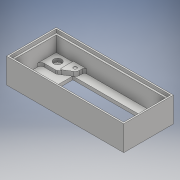
# Autodesk Inventor part: top
Saved by Autodesk Inventor 2018 (Build 220112000, 112)
## iProperties
Created: 2018-01-10
Part Number: top
Material: Generic
Document SubType Name: Modeling
Designer: gregg
Density: 1 g/cm^3
Appearance: Default
Author: gregg
Autodesk Inventor part; units mm, degrees
ref_plane "YZ Plane" through (0, 0, 0) normal (1, 0, 0) x (0, 1, 0)
ref_plane "XZ Plane" through (0, 0, 0) normal (0, 1, 0) x (-1, 0, 0)
ref_plane "XY Plane" through (0, 0, 0) normal (0, 0, 1) x (1, 0, 0)
sketch "Sketch1" plane through (0, 0, 0) normal (0, 0, 1) x (1, 0, 0)
  line L0 (0, 0) -> (100, 0)
  line L1 (100, 0) -> (100, 39)
  line L2 (100, 39) -> (0, 39)
  line L3 (0, 39) -> (0, 0)
  dimension "d45" = 100
  dimension "d46" = 39
  constraints: 8 end point, 2 parallel, 1 horizontal, 1 perpendicular
  measures "d45" distance of L1.end L2.end
  measures "d46" distance of L2.end L0.start
extrude "bottom" add sketch "Sketch1" along normal blind 3
sketch "Sketch5" plane through (0, 0, 0) normal (0, 0, -1) x (-1, 0, 0)
  line L0 (0, 0) -> (-100, 0) projected
  line L1 (0, 39) -> (0, 0) projected
  line L2 (-100, 39) -> (0, 39) projected
  line L3 (-100, 0) -> (-100, 39) projected
  line L4 (3, 42) -> (3, -3)
  line L5 (3, -3) -> (-103, -3)
  line L6 (-103, -3) -> (-103, 42)
  line L7 (-103, 42) -> (3, 42)
  dimension "d30" = 3
  constraints: 8 end point, 3 other
  measures "d30" distance between parallel lines of L2 L7
extrude "walls" add sketch "Sketch5" against normal blind 19.6
sketch "holes" plane through (0, 0, 0) normal (0, 0, 1) x (1, 0, 0)
  line L0 (0, 0) -> (100, 0) projected
  line L1 (100, 0) -> (100, 39) projected
  line L2 (100, 39) -> (0, 39) projected
  line L3 (0, 39) -> (0, 0) projected
  circle A0 centre (21.5, 34.5) radius 1.55 construction
  circle A1 centre (96.5, 34.5) radius 1.55 construction
  circle A2 centre (96.5, 3.5) radius 1.55 construction
  circle A3 centre (21.5, 3.5) radius 1.55 construction
  line L4 (21.5, 34.5) -> (21.5, 3.5) construction
  line L5 (21.5, 3.5) -> (96.5, 3.5) construction
  line L6 (96.5, 3.5) -> (96.5, 34.5) construction
  line L7 (96.5, 34.5) -> (21.5, 34.5) construction
  dimension "d33" = 3.1
  dimension "d34" = 75
  dimension "d35" = 31
  dimension "d50" = 3.5
  dimension "d51" = 3.5
  constraints: 8 end point, 4 centre point, 3 equal radius, 2 horizontal, 2 vertical
  measures "d33" diameter of A0
  measures "d34" distance of L6.end L4.start
  measures "d35" distance of L4.end L4.start
  measures "d50" distance from line of L1 L5.end
  measures "d51" distance from line of L0 L5.end
sketch "Sketch8" plane through (0, 0, 0) normal (0, 0, -1) x (-1, 0, 0)
  line L0 (-95, 6.3) -> (-23, 6.3)
  line L1 (-23, 6.3) -> (-23, 31)
  line L2 (-23, 31) -> (-95, 31)
  line L3 (-95, 31) -> (-95, 6.3)
  line L4 (3, -3) -> (-103, -3) projected
  line L5 (-96.5, 3.5) -> (-96.5, 34.5) construction
  line L6 (-21.5, 34.5) -> (-21.5, 3.5) construction
  point P0 (0, 0)
  dimension "d99" = 1.5
  dimension "d100" = 1.5
  dimension "d101" = 3.5
  dimension "d102" = 2.8
  constraints: 8 end point, 2 parallel, 1 horizontal, 1 perpendicular
  measures "d99" distance between parallel lines of L5 L3
  measures "d100" distance between parallel lines of L6 L1
  measures "d101" distance from line of L2 L5.end
  measures "d102" distance from line of L0 L5.start
extrude "display" cut sketch "Sketch8" along normal through all both and the other way through all
sketch "Sketch7" plane through (0, 0, 3) normal (0, 0, 1) x (1, 0, 0)
  circle A0 centre (96.5, 34.5) radius 1.55 construction
  circle A1 centre (21.5, 3.5) radius 1.55 construction
  circle A2 centre (21.5, 34.5) radius 1.55 construction
  arc A3 (23.4365, 31) -> (25.5, 34.5) centre (21.5, 34.5) ccw
  line L0 (15.5, 39) -> (27.5, 39)
  line L1 (0, 39) -> (100, 39) projected
  arc A4 (27.5, 39) -> (25.5, 37) centre (27.5, 37) ccw
  line L2 (25.5, 37) -> (25.5, 34.5)
  line L3 (16.3235, 0) -> (26.6765, 0)
  line L4 (23, 31) -> (95, 31) construction
  arc A5 (92.6921, 34.5) -> (96.7797, 30.7024) centre (96.5, 34.5) ccw
  line L5 (92.6921, 34.5) -> (92.6921, 36)
  arc A6 (92.6921, 36) -> (89.6921, 39) centre (89.6921, 36) ccw
  line L6 (100, 0) -> (100, 39) projected
  arc A7 (100, 27.7105) -> (96.7797, 30.7024) centre (97, 27.7105) ccw
  line L7 (100, 39) -> (0, 39) projected
  line L8 (89.6921, 39) -> (100, 39)
  line L9 (100, 39) -> (100, 27.7105)
  circle A8 centre (96.5, 3.5) radius 3.1765 construction
  line L10 (0, 0) -> (100, 0) projected
  arc A9 (90.3438, 0) -> (93.3339, 3.2429) centre (90.3438, 3) ccw construction
  arc A10 (96.7571, 6.6661) -> (100, 9.6562) centre (97, 9.6562) ccw construction
  line L11 (100, 9.6562) -> (100, 0)
  line L12 (100, 0) -> (90.3438, 0)
  line L13 (15.5, 39) -> (15.5, 27.8105)
  line L14 (17.0325, 26.964) -> (23.6299, 31.1142)
  line L15 (0, 0) -> (0, 39) projected
  arc A11 (15.5, 27.8105) -> (17.0325, 26.964) centre (16.5, 27.8105) ccw
  line L16 (100, 0) -> (0, 0) projected
  line L17 (96.5, 6.6765) -> (95, 6.6765) construction
  line L18 (95, 6.6765) -> (95, 6.3)
  line L19 (23, 6.3) -> (95, 6.3) projected
  line L20 (95, 6.3) -> (93.3235, 6.3)
  line L21 (93.3235, 6.3) -> (93.3235, 3.5) construction
  line L22 (91.8235, 6.3) -> (91.8235, 2)
  arc A12 (89.8235, 0) -> (91.8235, 2) centre (89.8235, 2) ccw
  line L23 (95, 8.1765) -> (98, 8.1765)
  arc A13 (98, 8.1765) -> (100, 10.1765) centre (98, 10.1765) ccw
  line L24 (100, 39) -> (100, 0) projected
  line L25 (95, 6.6765) -> (95, 8.1765)
  line L26 (95, 6.3) -> (95, 31) construction
  line L27 (95, 6.3) -> (23, 6.3) construction
  line L28 (26.5, 6.3) -> (26.5, 1.9199)
  arc A14 (26.5, 1.9199) -> (27.9398, 0) centre (28.5, 1.9199) ccw
  line L29 (23, 8.5) -> (18.5, 8.5)
  arc A15 (18.5, 8.5) -> (16.5, 6.5) centre (18.5, 6.5) ccw
  line L30 (16.5, 6.5) -> (16.5, 2)
  arc A16 (14.5, 0) -> (16.5, 2) centre (14.5, 2) ccw
  line L31 (23, 31) -> (23, 6.3) projected
  line L32 (23, 8.5) -> (23, 6.3)
  line L33 (23, 6.3) -> (26.5, 6.3)
  point P0 (15.5, 26)
  dimension "d54" = 8
  dimension "d61" = 3
  dimension "d62" = 3
  dimension "d65" = 3
  dimension "d66" = 3
  dimension "d81" = 15.5
  dimension "d82" = 13
  dimension "d83" = 1
  dimension "d103" = 1.5
  dimension "d104" = 1.5
  dimension "d105" = 2
  dimension "d106" = 2
  dimension "d117" = 2
  dimension "d118" = 5
  dimension "d119" = 5
  dimension "d120" = 2
  dimension "d121" = 2
  dimension "d122" = 2
  dimension "d123" = 5
  constraints: 44 end point, 34 point on circle, 26 tangent, 19 point on line, 14 centre point, 5 horizontal, 5 perpendicular, 5 vertical, 4 collinear, 3 coincident
  measures "d54" diameter of A3
  measures "d61" radius of A6
  measures "d62" radius of A7
  measures "d65" radius of A10
  measures "d66" radius of A9
  measures "d81" distance between parallel lines of L13 L15
  measures "d82" distance of point (15.5, 26) L13.start
  measures "d83" radius of A11
  measures "d103" distance between parallel lines of L23 L17
  measures "d104" distance between parallel lines of L22 L21
  measures "d105" radius of A12
  measures "d106" radius of A13
  measures "d117" radius of A4
  measures "d118" distance from line of L28 A1.centre
  measures "d119" distance from line of A1.centre L29
  measures "d120" radius of A14
  measures "d121" radius of A16
  measures "d122" radius of A15
  measures "d123" distance from line of A1.centre L30
extrude "Extrusion19" add sketch "Sketch7" along normal blind 3.8 contours L14 A11 L13 L0 A4 L2 A3 | L31 L19 L28 A14 L10 L3 A16 L30 A15 L29 | L1 L6 A7 A5 L5 A6 | L19 L18 L25 L23 A13 L6 L10 A12 L22
sketch "Sketch9" plane through (0, 0, 0) normal (0, 0, -1) x (-1, 0, 0)
  circle A0 centre (-21.5, 3.5) radius 1.55 construction
  circle A1 centre (-21.5, 34.5) radius 1.55 construction
  circle A2 centre (-21.5, 34.5) radius 3.1
  circle A3 centre (-21.5, 3.5) radius 3.1
  circle A4 centre (-96.5, 34.5) radius 1.55 construction
  circle A5 centre (-96.5, 3.5) radius 1.55 construction
  circle A6 centre (-96.5, 34.5) radius 3.1
  circle A7 centre (-96.5, 3.5) radius 3.1
  line L0 (-95, 6.3) -> (-95, 31) projected
  point P0 (0, 0)
  point P1 (-94.7478, 6.0573)
  point P2 (-95.3418, 6.3755)
  dimension "d57" = 6.2
  dimension "d58" = 6.2
  dimension "d109" = 6.2
  constraints: 4 centre point, 4 coincident, 2 point on circle, 1 equal radius
  measures "d57" diameter of A2
  measures "d58" diameter of A3
  measures "d109" diameter of A7
extrude "bolt holes" cut sketch "Sketch9" against normal blind 6.5
sketch "Sketch10" plane through (0, 0, 0) normal (0, 0, -1) x (-1, 0, 0)
  circle A0 centre (-96.5, 34.5) radius 1.55 projected
  circle A1 centre (-96.5, 3.5) radius 1.55 projected
  circle A2 centre (-21.5, 3.5) radius 1.55 projected
  circle A3 centre (-21.5, 34.5) radius 1.55 projected
  point P0 (0, 0)
extrude "holes screws" cut sketch "Sketch10" along normal through all both and the other way through all
sketch "Sketch11" plane through (96.5, 34.5, 6.5) normal (0, 0, -1) x (-1, 0, 0)
  circle A0 centre (75, 0) radius 1.55 projected
  circle A1 centre (75, 0) radius 3.1 projected
  circle A2 centre (75, -31) radius 3.1 projected
  circle A3 centre (0, -31) radius 1.55 projected
  circle A4 centre (0, -31) radius 3.1 projected
  circle A5 centre (0, 0) radius 3.1 projected
  point P0 (96.5, -34.5)
extrude "fill after hole" add sketch "Sketch11" along normal blind 0.6 contours A0 | A1 | A2 | A3 | A4 | A5
sketch "Sketch13" plane through (0, 0, 19.6) normal (0, 0, 1) x (1, 0, 0)
  line L0 (0, 0) -> (0, 39) projected
  line L1 (0, 39) -> (100, 39) projected
  line L2 (100, 39) -> (100, 0) projected
  line L3 (100, 0) -> (0, 0) projected
  line L4 (-3, 42) -> (-3, -3) projected
  line L5 (-3, -3) -> (103, -3) projected
  line L6 (103, -3) -> (103, 42) projected
  line L7 (103, 42) -> (-3, 42) projected
  line L8 (-1.7, 40.7) -> (-1.7, -1.7)
  line L9 (-1.7, -1.7) -> (101.7, -1.7)
  line L10 (101.7, -1.7) -> (101.7, 40.7)
  line L11 (101.7, 40.7) -> (-1.7, 40.7)
  dimension "d126" = 1.3
  dimension "d127" = 1.3
  dimension "d128" = 1.3
  dimension "d129" = 1.3
  constraints: 8 end point, 2 horizontal, 2 vertical
  measures "d126" distance between parallel lines of L9 L5
  measures "d127" distance between parallel lines of L6 L10
  measures "d128" distance between parallel lines of L7 L11
  measures "d129" distance between parallel lines of L4 L8
extrude "collar" add sketch "Sketch13" along normal blind 3 contours L7 L6 L5 L4
sketch "Sketch15" plane through (0, 0, 3) normal (0, 0, 1) x (1, 0, 0)
  line L0 (100, 39) -> (0, 39) projected
  line L1 (0, 39) -> (15.5, 39)
  line L2 (15.5, 39) -> (15.5, 27)
  line L3 (13.5, 25) -> (0, 25)
  line L4 (0, 25) -> (0, 39)
  line L5 (0, 0) -> (0, 39) projected
  arc A0 (3, 25) -> (0, 22) centre (3, 22) ccw
  line L6 (0, 25) -> (0, 22)
  arc A1 (13.5, 25) -> (15.5, 27) centre (13.5, 27) ccw
  line L7 (14.6154, 25.3399) -> (17.0325, 26.964)
  arc A2 (15.5, 27.8105) -> (17.0325, 26.964) centre (16.5, 27.8105) ccw projected
  point P0 (15.5, 39)
  point P1 (15.5, 25)
  dimension "d90" = 14
  dimension "d95" = 3
  dimension "d96" = 2
  constraints: 12 end point, 5 point on circle, 5 point on line, 5 tangent, 2 centre point, 2 parallel, 1 coincident, 1 collinear, 1 horizontal, 1 perpendicular
  measures "d90" distance of L1.end point (15.5, 25)
  measures "d95" radius of A0
  measures "d96" radius of A1
extrude "encoder standoff" add sketch "Sketch15" along normal blind 3
sketch "Sketch12" plane through (0, 0, 0) normal (0, 0, -1) x (-1, 0, 0)
  circle A0 centre (-7.75, 32.5) radius 3.6
  line L0 (0, 0) -> (0, 39) projected
  line L1 (-7.75, 32.5) -> (-15.5, 32.5) construction
  line L2 (-7.75, 32.5) -> (0, 32.5) construction
  line L3 (0, 39) -> (-100, 39) construction
  line L4 (0, 22) -> (0, 0) projected
  line L5 (-89.6921, 39) -> (-27.5, 39) projected
  line L6 (0, 22) -> (0, 39) projected
  line L7 (0, 39) -> (-15.5, 39) projected
  line L8 (-15.5, 39) -> (-15.5, 27.8105) projected
  line L9 (-15.5, 39) -> (-27.5, 39) projected
  line L10 (-89.6921, 39) -> (-100, 39) projected
  point P0 (-15.5, 39)
  dimension "d71" = 7.2
  dimension "d112" = 6.5
  constraints: 4 end point, 2 horizontal, 2 point on line, 1 centre point, 1 collinear
  measures "d71" diameter of A0
  measures "d112" distance between parallel lines of L7 L1
extrude "encoder hole" cut sketch "Sketch12" along normal through all both and the other way through all
sketch "Sketch14" plane through (0, 0, 0) normal (0, 0, -1) x (-1, 0, 0)
  circle A0 centre (-7.75, 32.5) radius 3.6 projected
  circle A1 centre (-7.75, 32.5) radius 7
  point P0 (0, 0)
  dimension "d87" = 14
  constraints: 1 centre point, 1 coincident
  measures "d87" diameter of A1
extrude "encoder nut" cut sketch "Sketch14" against normal blind 2.5
sketch "Sketch16" plane through (7.75, 32.5, 2.5) normal (0, 0, -1) x (-1, 0, 0)
  circle A0 centre (0, 0) radius 3.6 projected
  point P0 (7.75, -32.5)
extrude "encoder fill before hole" add sketch "Sketch16" against normal blind 0.6
sketch "Sketch18" plane through (0, 0, 6.8) normal (0, 0, 1) x (1, 0, 0)
  circle A0 centre (21.5, 34.5) radius 1.55 projected
  line L0 (15.5, 39) -> (15.5, 27.8105) projected
  arc A1 (15.5, 27.8105) -> (17.0325, 26.964) centre (16.5, 27.8105) ccw projected
  line L1 (17.0325, 26.964) -> (23.6299, 31.1142) projected
  arc A2 (23.6299, 31.1142) -> (25.5, 34.5) centre (21.5, 34.5) ccw projected
  line L2 (25.5, 34.5) -> (25.5, 37) projected
  arc A3 (27.5, 39) -> (25.5, 37) centre (27.5, 37) ccw projected
  line L3 (15.5, 39) -> (27.5, 39) projected
  circle A4 centre (21.5, 3.5) radius 1.55 projected
  arc A5 (14.5, 0) -> (16.5, 2) centre (14.5, 2) ccw projected
  line L4 (27.9398, 0) -> (14.5, 0) projected
  arc A6 (26.5, 1.9199) -> (27.9398, 0) centre (28.5, 1.9199) ccw projected
  line L5 (26.5, 6.3) -> (26.5, 1.9199) projected
  line L6 (23, 6.3) -> (26.5, 6.3) projected
  line L7 (23, 8.5) -> (23, 6.3) projected
  line L8 (18.5, 8.5) -> (23, 8.5) projected
  arc A7 (18.5, 8.5) -> (16.5, 6.5) centre (18.5, 6.5) ccw projected
  line L9 (16.5, 2) -> (16.5, 6.5) projected
  circle A8 centre (96.5, 3.5) radius 1.55 projected
  line L10 (100, 0) -> (89.8235, 0) projected
  line L11 (100, 10.1765) -> (100, 0) projected
  arc A9 (98, 8.1765) -> (100, 10.1765) centre (98, 10.1765) ccw projected
  line L12 (95, 8.1765) -> (98, 8.1765) projected
  line L13 (95, 6.3) -> (95, 8.1765) projected
  line L14 (91.8235, 6.3) -> (95, 6.3) projected
  line L15 (91.8235, 2) -> (91.8235, 6.3) projected
  arc A10 (89.8235, 0) -> (91.8235, 2) centre (89.8235, 2) ccw projected
  circle A11 centre (96.5, 34.5) radius 1.55 projected
  arc A12 (92.6921, 36) -> (89.6921, 39) centre (89.6921, 36) ccw projected
  line L16 (92.6921, 34.5) -> (92.6921, 36) projected
  arc A13 (92.6921, 34.5) -> (96.7797, 30.7024) centre (96.5, 34.5) ccw projected
  arc A14 (100, 27.7105) -> (96.7797, 30.7024) centre (97, 27.7105) ccw projected
  line L17 (100, 39) -> (100, 27.7105) projected
  line L18 (89.6921, 39) -> (100, 39) projected
  point P0 (0, 0)
extrude "Extrusion21" add sketch "Sketch18" along normal blind 0.1
body "Solid1"
